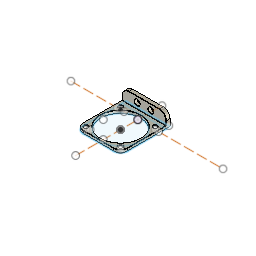
Fan NF-A6x25 support 4020 profile v1 (Autodesk Fusion 360 design; units mm, degrees)
Autodesk Fusion 360 part; units mm, degrees
note: some values were not read from the file. Set by a fixed rule: which sketch regions a step uses; the direction of a hole.
sketch "Sketch1" plane through (0, 0, 0) normal (0, 0, 1) x (1, 0, 0)
  line L0 (30, 15) -> (-30, 15)
  line L1 (-32, 15) -> (32, 15)
  line L2 (32, 9) -> (-32, 9)
  line L3 (-96.8197, 0) -> (-30, 0) construction
  line L4 (30, 0) -> (123.3846, 0) construction
  circle A0 centre (0, -25) radius 29
  line L5 (-20, 0) -> (-14.6969, 0) construction
  line L6 (-32, -47) -> (-32, 15)
  line L7 (0, 35) -> (0, -90) construction
  line L8 (-22, -57) -> (22, -57)
  line L9 (32, -47) -> (32, 15)
  arc A1 (-32, -47) -> (-22, -57) centre (-22, -47) ccw
  arc A2 (22, -57) -> (32, -47) centre (22, -47) ccw
  point P0 (-25, 0)
  point P1 (-25, -25)
  point P2 (0, -25)
  point P3 (-25, -50)
  point P4 (0, -50)
  point P5 (25, -50)
  point P6 (25, 0)
  dimension "d1" = 25
  dimension "d12" = 50
  dimension "d13" = -50
  dimension "d14" = 58
  dimension "d25" = 10
  constraint horizontal L3
  constraint coincident P0 L3
  constraint horizontal L0
  constraint horizontal L1
  constraint horizontal L2
  constraint collinear L3 L5
  constraint collinear L4 L5
  constraint coincident P2 A0.centre
  constraint coincident A0 L5.end
  constraint perpendicular L3 L6
  constraint coincident L0.end L1
  constraint coincident L6 L2.end
  constraint perpendicular L1 L7
  constraint horizontal L8
  constraint symmetric P0 L7 P6
  constraint symmetric P3 L7 P5
  constraint symmetric L1.start L7 L1.end
  constraint coincident L9 L2.start
  constraint tangent L6 A1
  constraint tangent L8 A1
  constraint tangent L8 A2
  constraint tangent L9 A2
  constraint equal A1 A2
  measures "d1" distance of origin P0
  measures "d14" diameter of A0
  measures "d25" radius of A1
extrude "Extrude1" add sketch "Sketch1" along normal blind 6 contours L0 L1 L2 L6 L9
extrude "Extrude2" add sketch "Sketch1" along normal blind 20 contours L0 L1 L2 L6 L9
extrude "Extrude3" add sketch "Sketch1" along normal blind 4 contours L2 L6 L8 L9 A1 A2
hole "Hole1" at (-25, -50, 0) at (25, -50, 0) at (25, 0, 0) at (-25, 0, 0) direction (0, 0, 1) diameter 5.5 depth 14 tip angle 118
sketch "Sketch2" plane through (0, 9, 0) normal (0, -1, 0) x (1, 0, 0)
  line L0 (-32, 4) -> (32, 4)
  line L1 (32, 4) -> (32, 20)
  line L2 (32, 20) -> (-32, 20)
  line L3 (-32, 20) -> (-32, 4)
  line L4 (0, 37.8126) -> (0, -29.4999) construction
  point P0 (-10, 12)
  point P1 (10, 12)
  dimension "d26" = 10
  constraint perpendicular L2 L4
  constraint symmetric P0 L4 P1
  measures "d26" distance of P0 L4
hole "Hole2" at (-10, 9, 12) at (10, 9, 12) direction (0, 1, 0) diameter 4.5 depth 14 tip angle 118 counterbore diameter 8 counterbore depth 4
fillet "Fillet1" radius 10 2 edges at (-32, 12, 20) (32, 12, 20)
fillet "Fillet2" radius 0.4 10 faces at (-0.7224, 7.3063, 4) (-7.3333, 11, 20) (22.9506, 11, 19.9547) (32, 13, 4.6667) (30.1458, -52.8006, 2.6667) (-7.3333, -57, 1.3333) (-31.7181, -49.3576, 2.6667) (-32, 13, 4.6667) (-31.9887, 13, 10.4758) (25.9078, 9, 8.1795)
